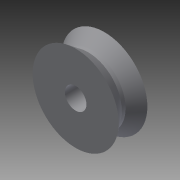
# Autodesk Inventor part: bearing V groove 12mm
Saved by Autodesk Inventor 2013 SP2 (Build 170200200, 200)
## iProperties
Created: 2017-05-17
Part Number: bearing V groove 12mm
Material: Generic
Document SubType Name: Modeling
Designer: Herman de Vries
Density: 1 g/cm^3
Mass: 0.320442 g
Surface Area: 4.1469 cm^2
Volume: 0.320442 cm^3
Author: Herman de Vries
Autodesk Inventor part; units mm, degrees
ref_plane "YZ Plane" through (0, 0, 0) normal (1, 0, 0) x (0, 1, 0)
ref_plane "XZ Plane" through (0, 0, 0) normal (0, 1, 0) x (-1, 0, 0)
ref_plane "XY Plane" through (0, 0, 0) normal (0, 0, 1) x (1, 0, 0)
sketch "Sketch1" plane through (0, 0, 0) normal (0, 0, 1) x (1, 0, 0)
  line L0 (1.5, 0) -> (6, 0)
  line L1 (6, 0) -> (6, 4) construction
  line L2 (6, 4) -> (1.5, 4)
  line L3 (1.5, 4) -> (1.5, 0)
  line L4 (6, 4) -> (4.5, 2)
  line L5 (4.5, 2) -> (6.0886, -0.1181)
  line L6 (0, 0) -> (0, 6.0254) construction
  line L7 (4.7, 2.2667) -> (3.3665, 2.2667)
  line L8 (3.3665, 2.2667) -> (3.3665, 1.7333)
  line L9 (3.3665, 1.7333) -> (4.7, 1.7333)
  line L10 (4.7, 1.7333) -> (4.7, 2.2667)
  point P0 (6, 2)
  point P1 (4.7, 2)
  dimension "d0" = 1.5
  dimension "d1" = 4
  dimension "d2" = 6
  dimension "d3" = 1.5
  dimension "d5" = 0.2
  constraints: 22 end point, 5 parallel, 3 horizontal alignment, 2 horizontal, 2 midpoint, 2 perpendicular, 2 point on line
  measures "d0" distance from line of L3 L6.start
  measures "d1" distance of L0.end L1.end
  measures "d2" distance from line of L1 L6.start
  measures "d3" distance from line of L1 L4.end
  measures "d5" distance from line of L10 L4.end
revolve "Revolution1" add sketch "Sketch1" angle 360 about axis through (0, 0, 0) along (0, 1, 0)
body "Solid1"
